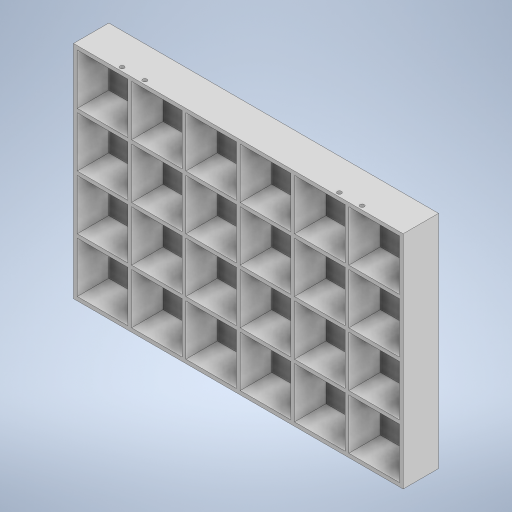
# Autodesk Inventor part: RatPelletBox_v03
Saved by Autodesk Inventor 2023.5 (Build 275446000, 446)
## iProperties
Created: 2025-06-19
Part Number: RatPelletBox_v03
Material: Generic
Document SubType Name: Modeling
Designer: Akramilab
Density: 1 g/cm^3
Appearance: Default
Author: Akramilab
Autodesk Inventor part; units mm, degrees
ref_plane "YZ Plane" through (0, 0, 0) normal (1, 0, 0) x (0, 1, 0)
ref_plane "XZ Plane" through (0, 0, 0) normal (0, 1, 0) x (-1, 0, 0)
ref_plane "XY Plane" through (0, 0, 0) normal (0, 0, 1) x (1, 0, 0)
sketch "Sketch1" plane through (0, 0, 0) normal (0, 0, 1) x (1, 0, 0)
  line L0 (-130.5, -87.5) -> (130.5, -87.5)
  line L1 (130.5, -87.5) -> (130.5, 87.5)
  line L2 (130.5, 87.5) -> (-130.5, 87.5)
  line L3 (-130.5, 87.5) -> (-130.5, -87.5)
  line L4 (-130.5, -87.5) -> (130.5, 87.5) construction
  line L5 (130.5, -87.5) -> (-130.5, 87.5) construction
  point P0 (0, 0)
  dimension "d0" = 261
  dimension "d1" = 175
  constraints: 12 end point, 2 midpoint, 2 parallel, 1 horizontal, 1 perpendicular
  measures "d0" distance of L1.end L2.end
  measures "d1" distance of L0.end L1.end
extrude "Extrusion1" add sketch "Sketch1" along normal blind 28
sketch "Sketch2" plane through (0, 0, 28) normal (0, 0, 1) x (1, 0, 0)
  line L0 (-127.5, 84.5) -> (-87.5, 84.5)
  line L1 (-87.5, 84.5) -> (-87.5, 44.5)
  line L2 (-87.5, 44.5) -> (-127.5, 44.5)
  line L3 (-127.5, 44.5) -> (-127.5, 84.5)
  line L4 (-127.5, 84.5) -> (-87.5, 44.5) construction
  line L5 (-87.5, 84.5) -> (-127.5, 44.5) construction
  line L6 (130.5, 87.5) -> (-130.5, 87.5) projected
  line L7 (-130.5, 87.5) -> (-130.5, -87.5) projected
  line L8 (-84.5, 84.5) -> (-44.5, 84.5)
  line L9 (-44.5, 84.5) -> (-44.5, 44.5)
  line L10 (-44.5, 44.5) -> (-84.5, 44.5)
  line L11 (-84.5, 44.5) -> (-84.5, 84.5)
  line L12 (-84.5, 84.5) -> (-44.5, 44.5) construction
  line L13 (-44.5, 84.5) -> (-84.5, 44.5) construction
  line L14 (-41.5, 84.5) -> (-1.5, 84.5)
  line L15 (-1.5, 84.5) -> (-1.5, 44.5)
  line L16 (-1.5, 44.5) -> (-41.5, 44.5)
  line L17 (-41.5, 44.5) -> (-41.5, 84.5)
  line L18 (-41.5, 84.5) -> (-1.5, 44.5) construction
  line L19 (-1.5, 84.5) -> (-41.5, 44.5) construction
  line L20 (1.5, 84.5) -> (41.5, 84.5)
  line L21 (41.5, 84.5) -> (41.5, 44.5)
  line L22 (41.5, 44.5) -> (1.5, 44.5)
  line L23 (1.5, 44.5) -> (1.5, 84.5)
  line L24 (1.5, 84.5) -> (41.5, 44.5) construction
  line L25 (41.5, 84.5) -> (1.5, 44.5) construction
  line L26 (44.5, 84.5) -> (84.5, 84.5)
  line L27 (84.5, 84.5) -> (84.5, 44.5)
  line L28 (84.5, 44.5) -> (44.5, 44.5)
  line L29 (44.5, 44.5) -> (44.5, 84.5)
  line L30 (44.5, 84.5) -> (84.5, 44.5) construction
  line L31 (84.5, 84.5) -> (44.5, 44.5) construction
  line L32 (-127.5, 41.5) -> (-87.5, 41.5)
  line L33 (-87.5, 41.5) -> (-87.5, 1.5)
  line L34 (-87.5, 1.5) -> (-127.5, 1.5)
  line L35 (-127.5, 1.5) -> (-127.5, 41.5)
  line L36 (-127.5, 41.5) -> (-87.5, 1.5) construction
  line L37 (-87.5, 41.5) -> (-127.5, 1.5) construction
  line L38 (-84.5, 41.5) -> (-44.5, 41.5)
  line L39 (-44.5, 41.5) -> (-44.5, 1.5)
  line L40 (-44.5, 1.5) -> (-84.5, 1.5)
  line L41 (-84.5, 1.5) -> (-84.5, 41.5)
  line L42 (-84.5, 41.5) -> (-44.5, 1.5) construction
  line L43 (-44.5, 41.5) -> (-84.5, 1.5) construction
  line L44 (-41.5, 41.5) -> (-1.5, 41.5)
  line L45 (-1.5, 41.5) -> (-1.5, 1.5)
  line L46 (-1.5, 1.5) -> (-41.5, 1.5)
  line L47 (-41.5, 1.5) -> (-41.5, 41.5)
  line L48 (-41.5, 41.5) -> (-1.5, 1.5) construction
  line L49 (-1.5, 41.5) -> (-41.5, 1.5) construction
  line L50 (1.5, 41.5) -> (41.5, 41.5)
  line L51 (41.5, 41.5) -> (41.5, 1.5)
  line L52 (41.5, 1.5) -> (1.5, 1.5)
  line L53 (1.5, 1.5) -> (1.5, 41.5)
  line L54 (1.5, 41.5) -> (41.5, 1.5) construction
  line L55 (41.5, 41.5) -> (1.5, 1.5) construction
  line L56 (44.5, 41.5) -> (84.5, 41.5)
  line L57 (84.5, 41.5) -> (84.5, 1.5)
  line L58 (84.5, 1.5) -> (44.5, 1.5)
  line L59 (44.5, 1.5) -> (44.5, 41.5)
  line L60 (44.5, 41.5) -> (84.5, 1.5) construction
  line L61 (84.5, 41.5) -> (44.5, 1.5) construction
  line L62 (-127.5, -1.5) -> (-87.5, -1.5)
  line L63 (-87.5, -1.5) -> (-87.5, -41.5)
  line L64 (-87.5, -41.5) -> (-127.5, -41.5)
  line L65 (-127.5, -41.5) -> (-127.5, -1.5)
  line L66 (-127.5, -1.5) -> (-87.5, -41.5) construction
  line L67 (-87.5, -1.5) -> (-127.5, -41.5) construction
  line L68 (-84.5, -1.5) -> (-44.5, -1.5)
  line L69 (-44.5, -1.5) -> (-44.5, -41.5)
  line L70 (-44.5, -41.5) -> (-84.5, -41.5)
  line L71 (-84.5, -41.5) -> (-84.5, -1.5)
  line L72 (-84.5, -1.5) -> (-44.5, -41.5) construction
  line L73 (-44.5, -1.5) -> (-84.5, -41.5) construction
  line L74 (-41.5, -1.5) -> (-1.5, -1.5)
  line L75 (-1.5, -1.5) -> (-1.5, -41.5)
  line L76 (-1.5, -41.5) -> (-41.5, -41.5)
  line L77 (-41.5, -41.5) -> (-41.5, -1.5)
  line L78 (-41.5, -1.5) -> (-1.5, -41.5) construction
  line L79 (-1.5, -1.5) -> (-41.5, -41.5) construction
  line L80 (1.5, -1.5) -> (41.5, -1.5)
  line L81 (41.5, -1.5) -> (41.5, -41.5)
  line L82 (41.5, -41.5) -> (1.5, -41.5)
  line L83 (1.5, -41.5) -> (1.5, -1.5)
  line L84 (1.5, -1.5) -> (41.5, -41.5) construction
  line L85 (41.5, -1.5) -> (1.5, -41.5) construction
  line L86 (44.5, -1.5) -> (84.5, -1.5)
  line L87 (84.5, -1.5) -> (84.5, -41.5)
  line L88 (84.5, -41.5) -> (44.5, -41.5)
  line L89 (44.5, -41.5) -> (44.5, -1.5)
  line L90 (44.5, -1.5) -> (84.5, -41.5) construction
  line L91 (84.5, -1.5) -> (44.5, -41.5) construction
  line L92 (-127.5, -44.5) -> (-87.5, -44.5)
  line L93 (-87.5, -44.5) -> (-87.5, -84.5)
  line L94 (-87.5, -84.5) -> (-127.5, -84.5)
  line L95 (-127.5, -84.5) -> (-127.5, -44.5)
  line L96 (-127.5, -44.5) -> (-87.5, -84.5) construction
  line L97 (-87.5, -44.5) -> (-127.5, -84.5) construction
  line L98 (-84.5, -44.5) -> (-44.5, -44.5)
  line L99 (-44.5, -44.5) -> (-44.5, -84.5)
  line L100 (-44.5, -84.5) -> (-84.5, -84.5)
  line L101 (-84.5, -84.5) -> (-84.5, -44.5)
  line L102 (-84.5, -44.5) -> (-44.5, -84.5) construction
  line L103 (-44.5, -44.5) -> (-84.5, -84.5) construction
  line L104 (-41.5, -44.5) -> (-1.5, -44.5)
  line L105 (-1.5, -44.5) -> (-1.5, -84.5)
  line L106 (-1.5, -84.5) -> (-41.5, -84.5)
  line L107 (-41.5, -84.5) -> (-41.5, -44.5)
  line L108 (-41.5, -44.5) -> (-1.5, -84.5) construction
  line L109 (-1.5, -44.5) -> (-41.5, -84.5) construction
  line L110 (1.5, -44.5) -> (41.5, -44.5)
  line L111 (41.5, -44.5) -> (41.5, -84.5)
  line L112 (41.5, -84.5) -> (1.5, -84.5)
  line L113 (1.5, -84.5) -> (1.5, -44.5)
  line L114 (1.5, -44.5) -> (41.5, -84.5) construction
  line L115 (41.5, -44.5) -> (1.5, -84.5) construction
  line L116 (44.5, -44.5) -> (84.5, -44.5)
  line L117 (84.5, -44.5) -> (84.5, -84.5)
  line L118 (84.5, -84.5) -> (44.5, -84.5)
  line L119 (44.5, -84.5) -> (44.5, -44.5)
  line L120 (44.5, -44.5) -> (84.5, -84.5) construction
  line L121 (84.5, -44.5) -> (44.5, -84.5) construction
  line L122 (87.5, 84.5) -> (127.5, 84.5)
  line L123 (127.5, 84.5) -> (127.5, 44.5)
  line L124 (127.5, 44.5) -> (87.5, 44.5)
  line L125 (87.5, 44.5) -> (87.5, 84.5)
  line L126 (87.5, 84.5) -> (127.5, 44.5) construction
  line L127 (127.5, 84.5) -> (87.5, 44.5) construction
  line L128 (87.5, 41.5) -> (127.5, 41.5)
  line L129 (127.5, 41.5) -> (127.5, 1.5)
  line L130 (127.5, 1.5) -> (87.5, 1.5)
  line L131 (87.5, 1.5) -> (87.5, 41.5)
  line L132 (87.5, 41.5) -> (127.5, 1.5) construction
  line L133 (127.5, 41.5) -> (87.5, 1.5) construction
  line L134 (87.5, -1.5) -> (127.5, -1.5)
  line L135 (127.5, -1.5) -> (127.5, -41.5)
  line L136 (127.5, -41.5) -> (87.5, -41.5)
  line L137 (87.5, -41.5) -> (87.5, -1.5)
  line L138 (87.5, -1.5) -> (127.5, -41.5) construction
  line L139 (127.5, -1.5) -> (87.5, -41.5) construction
  line L140 (87.5, -44.5) -> (127.5, -44.5)
  line L141 (127.5, -44.5) -> (127.5, -84.5)
  line L142 (127.5, -84.5) -> (87.5, -84.5)
  line L143 (87.5, -84.5) -> (87.5, -44.5)
  line L144 (87.5, -44.5) -> (127.5, -84.5) construction
  line L145 (127.5, -44.5) -> (87.5, -84.5) construction
  point P0 (0, 0)
  point P1 (-107.5, 64.5)
  point P2 (-64.5, 64.5)
  point P3 (-21.5, 64.5)
  point P4 (21.5, 64.5)
  point P5 (64.5, 64.5)
  point P6 (-107.5, 21.5)
  point P7 (-64.5, 21.5)
  point P8 (-21.5, 21.5)
  point P9 (21.5, 21.5)
  point P10 (64.5, 21.5)
  point P11 (-107.5, -21.5)
  point P12 (-64.5, -21.5)
  point P13 (-21.5, -21.5)
  point P14 (21.5, -21.5)
  point P15 (64.5, -21.5)
  point P16 (-107.5, -64.5)
  point P17 (-64.5, -64.5)
  point P18 (-21.5, -64.5)
  point P19 (21.5, -64.5)
  point P20 (64.5, -64.5)
  point P21 (107.5, 64.5)
  point P22 (107.5, 21.5)
  point P23 (107.5, -21.5)
  point P24 (107.5, -64.5)
  dimension "d4" = 40
  dimension "d5" = 3
  dimension "d6" = 3
  dimension "d7" = 40
  dimension "d10" = 43
  dimension "d13" = 43
  constraints: 288 end point, 2 collinear, 2 horizontal, 2 midpoint, 2 parallel, 1 perpendicular, 1 vertical, 251 other
  measures "d4" distance of L0.start L0.end
  measures "d5" distance between parallel lines of L6 L0
  measures "d6" distance between parallel lines of L7 L3
  measures "d7" distance of L0.end L1.end
  measures "d10" distance of L0.start L8.start
  measures "d13" distance of L0.start L32.start
extrude "Extrusion2" cut sketch "Sketch2" against normal blind 25
sketch "Sketch3" plane through (-130.5, 87.5, 0) normal (0, 1, 0) x (1, 0, 0)
  line L0 (46, -28) -> (46, -3) construction
  line L1 (43, -28) -> (43, -3) construction
  line L2 (43, -28) -> (43, -3) projected
  line L3 (43, -25) -> (46, -25) construction
  line L4 (46, -28) -> (46, -3) projected
  line L5 (261, -28) -> (0, -28) projected
  circle A0 centre (53.5, -25) radius 1.65
  circle A1 centre (35.5, -25) radius 1.65
  line L6 (172, -28) -> (172, -3) construction
  line L7 (175, -28) -> (175, -3) construction
  circle A2 centre (225.5, -25) radius 1.65
  circle A3 centre (207.5, -25) radius 1.65
  line L8 (261, 0) -> (261, -28) projected
  point P0 (130.5, 0)
  point P1 (44.5, -25)
  dimension "d20" = 3
  dimension "d21" = 3.3
  dimension "d22" = 9
  dimension "d23" = 3.3
  dimension "d24" = 9
  dimension "d25" = 3.3
  dimension "d31" = 3.3
  dimension "d35" = 18
  dimension "d36" = 35.5
  constraints: 4 centre point, 4 point on line, 2 end point, 1 midpoint, 1 perpendicular
  measures "d20" distance from line of L5 point (44.5, -25)
  measures "d21" diameter of A0
  measures "d22" distance of A0.centre point (44.5, -25)
  measures "d23" diameter of A1
  measures "d24" distance of A1.centre point (44.5, -25)
  measures "d25" diameter of A2
  measures "d31" diameter of A3
  measures "d35" distance of A2.centre A3.centre
  measures "d36" distance from line of A2.centre L8
extrude "Extrusion3" cut sketch "Sketch3" against normal blind 10
equation "\"d0\" = box_length"
equation "\"d1\" = box_width"
equation "\"d2\" = hole_height + wall"
equation "\"d4\" = hole"
equation "\"d5\" = wall"
equation "\"d6\" = wall"
equation "\"d7\" = hole"
equation "\"d10\" = hole + wall"
equation "\"d13\" = hole + wall"
equation "\"d16\" = hole_height"
equation "\"d23\" = d21"
equation "\"d24\" = d22"
equation "\"d25\" = d21"
equation "\"d31\" = d25"
equation "\"hole\" = 40"
equation "\"wall\" = 3"
equation "\"hole_height\" = 25"
equation "\"box_length\" = 261"
equation "\"box_width\" = 175"
body "Solid1"
